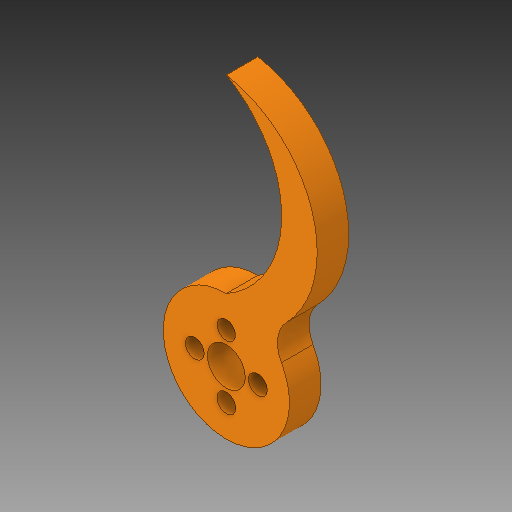
# Autodesk Inventor part: claw beta
Saved by Autodesk Inventor 2017 (Build 210142000, 142)
## iProperties
Created: 2018-01-13
Part Number: claw beta
Material: Generic
Document SubType Name: Modeling
Designer: Delta
Density: 1 g/cm^3
Appearance: Orange
Mass: 4.41121 g
Surface Area: 29.1303 cm^2
Volume: 4.41121 cm^3
Author: Delta
Autodesk Inventor part; units mm, degrees
ref_plane "YZ Plane" through (0, 0, 0) normal (1, 0, 0) x (0, 1, 0)
ref_plane "XZ Plane" through (0, 0, 0) normal (0, 1, 0) x (-1, 0, 0)
ref_plane "XY Plane" through (0, 0, 0) normal (0, 0, 1) x (1, 0, 0)
sketch "Sketch1" plane through (0, 0, 0) normal (0, 0, 1) x (1, 0, 0)
  circle A0 centre (0, 0) radius 12.7
  dimension "d0" = 25.4
  constraints: 1 centre point, 1 coincident
  measures "d0" diameter of A0
extrude "Extrusion1" add sketch "Sketch1" along normal blind 6.35
sketch "Sketch2" plane through (0, 0, 6.35) normal (0, 0, 1) x (1, 0, 0)
  circle A0 centre (0, 0) radius 3.81
  dimension "d3" = 7.62
  constraints: 1 centre point, 1 coincident
  measures "d3" diameter of A0
extrude "Extrusion2" cut sketch "Sketch2" against normal blind 6.35
sketch "Sketch3" plane through (0, 0, 6.35) normal (0, 0, 1) x (1, 0, 0)
  circle A0 centre (0, 6.35) radius 1.8415
  point P0 (0, 0)
  dimension "d6" = 3.683
  dimension "d7" = 6.35
  constraints: 1 centre point
  measures "d6" diameter of A0
  measures "d7" distance of A0.centre point (0, 0)
extrude "Extrusion3" cut sketch "Sketch3" against normal blind 6.35
sketch "Sketch4" plane through (0, 0, 6.35) normal (0, 0, 1) x (1, 0, 0)
  circle A0 centre (6.35, 0) radius 1.905
  circle A1 centre (0, -6.35) radius 1.905
  circle A2 centre (-6.35, 0) radius 1.905
  point P0 (0, 0)
  dimension "d10" = 3.81
  dimension "d11" = 3.81
  dimension "d12" = 3.81
  dimension "d13" = 6.35
  dimension "d14" = 6.35
  dimension "d15" = 6.35
  constraints: 3 centre point
  measures "d10" diameter of A0
  measures "d11" diameter of A1
  measures "d12" diameter of A2
  measures "d13" distance of A1.centre point (0, 0)
  measures "d14" distance of A0.centre point (0, 0)
  measures "d15" distance of A2.centre point (0, 0)
extrude "Extrusion4" cut sketch "Sketch4" against normal blind 6.35
sketch "Sketch5" plane through (0, 0, 6.35) normal (0, 0, 1) x (1, 0, 0)
  circle A0 centre (0, 0) radius 12.7 projected
  arc A1 (0, 12.7) -> (0, 50.8) centre (-10.7218, 31.75) ccw
  line L0 (0, 12.7) -> (0, 50.8) construction
  line L1 (0, 12.7) -> (38.1, 12.7) construction
  arc A2 (7.3073, 9.9507) -> (0, 50.8) centre (-3.7987, 29.0422) ccw
  arc A3 (0, 12.7) -> (7.3073, 9.9507) centre (4.4505, 13.4432) ccw
  dimension "d18" = 38.1
  dimension "d19" = 90
  constraints: 6 point on circle, 4 end point, 3 centre point, 1 horizontal, 1 perpendicular, 1 vertical alignment, 1 other
  measures "d18" distance of L0.start L0.end
  measures "d19" angle of L1 L0
extrude "Extrusion5" add sketch "Sketch5" against normal blind 6.35 contours A1 A2 A0 | A0 A2 A3 picked at (3.7894, 11.0049)
fillet "Fillet1" radius 6.35 1 edges at (7.6377, 10.1467, 3.175)
body "Solid1"
